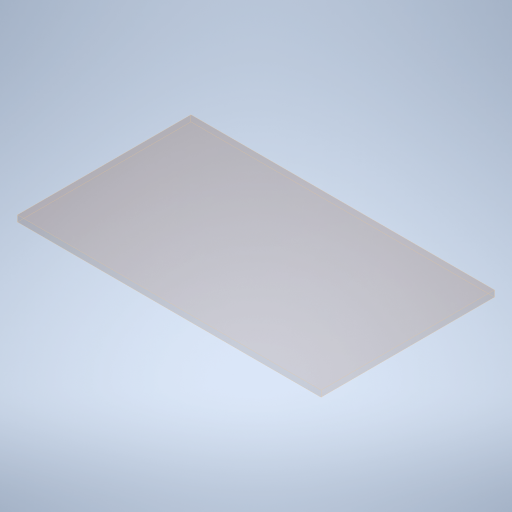
# Autodesk Inventor part: swerve_polyc
Saved by Autodesk Inventor 2024 (Build 280153000, 153)
## iProperties
Created: 2023-10-09
Part Number: swerve_polyc
Material: Polycarbonate, Smoke
Document SubType Name: Modeling
Designer: s137416
Density: 1.2 g/cm^3
Appearance: Polycarbonate - Smoked
Author: s137416
Autodesk Inventor part; units mm, degrees
ref_plane "YZ Plane" through (0, 0, 0) normal (1, 0, 0) x (0, 1, 0)
ref_plane "XZ Plane" through (0, 0, 0) normal (0, 1, 0) x (-1, 0, 0)
ref_plane "XY Plane" through (0, 0, 0) normal (0, 0, 1) x (1, 0, 0)
sketch "Sketch1" plane through (0, 0, 0) normal (0, 1, 0) x (-1, 0, 0)
  line L0 (9.9274, 340.0419) -> (-612.3726, 340.0419)
  line L1 (-612.3726, 340.0419) -> (-612.3726, -15.5581)
  line L2 (-612.3726, -15.5581) -> (9.9274, -15.5581)
  line L3 (9.9274, -15.5581) -> (9.9274, 340.0419)
  point P0 (0, 0)
  dimension "d0" = 622.3
  dimension "d1" = 355.6
  constraints: 8 end point, 2 parallel, 1 horizontal, 1 perpendicular
  measures "d0" distance of L2.end L1.end
  measures "d1" distance of L2.end L0.start
extrude "Extrusion1" add sketch "Sketch1" along normal blind 12.7
body "Solid1"
